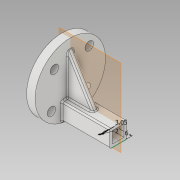
# Autodesk Inventor part: Motor Mount v1
Saved by Autodesk Inventor 2021 (Build 250183000, 183)
## iProperties
Created: 2019-01-09
Part Number: Motor Mount v1
Material: ABS Plastic
Document SubType Name: Modeling
Designer: Kanenas
Density: 1.06 g/cm^3
Appearance: Smooth - White
Mass: 1.86901 g
Surface Area: 21.0001 cm^2
Volume: 1.76322 cm^3
Author: Kanenas
Autodesk Inventor part; units mm, degrees
ref_plane "YZ Plane" through (0, 0, 0) normal (1, 0, 0) x (0, 1, 0)
ref_plane "XZ Plane" through (0, 0, 0) normal (0, 1, 0) x (-1, 0, 0)
sketch "Sketch1" plane through (0, 0, 0) normal (1, 0, 0) x (0, 1, 0)
  line L0 (3.05, 3.05) -> (-3.05, 3.05)
  line L1 (-3.05, 3.05) -> (-3.05, -3.05)
  line L2 (-3.05, -3.05) -> (3.05, -3.05)
  line L3 (3.05, -3.05) -> (3.05, 3.05)
  line L4 (3.05, 3.05) -> (-3.05, -3.05) construction
  line L5 (-3.05, 3.05) -> (3.05, -3.05) construction
  line L6 (2.05, 2.05) -> (-2.05, 2.05)
  line L7 (-2.05, 2.05) -> (-2.05, -2.05)
  line L8 (-2.05, -2.05) -> (2.05, -2.05)
  line L9 (2.05, -2.05) -> (2.05, 2.05)
  line L10 (2.05, 2.05) -> (-2.05, -2.05) construction
  line L11 (-2.05, 2.05) -> (2.05, -2.05) construction
  point P0 (0, 0)
  dimension "d0" = 6.1
  dimension "d1" = 6.1
  dimension "d2" = 4.1
  dimension "d3" = 4.1
  constraints: 24 end point, 4 midpoint, 4 parallel, 2 horizontal, 2 perpendicular
  measures "d0" distance of L2.end L0.start
  measures "d1" distance of L1.end L2.end
  measures "d2" distance of L8.end L6.start
  measures "d3" distance of L7.end L8.end
extrude "Extrusion1" add sketch "Sketch1" along normal blind 20
sketch "Sketch2" plane through (0, 0, 0) normal (-1, 0, 0) x (0, 0, 1)
  circle A0 centre (0, 8.5) radius 12.5
  line L0 (3.05, -3.05) -> (-3.05, -3.05) projected
  line L1 (3.05, -3.05) -> (-3.05, -3.05) projected
  point P0 (0, 0)
  dimension "d6" = 25
  dimension "d8" = 0
  dimension "d63" = 8.5
  constraints: 1 centre point
  measures "d6" diameter of A0
  measures "d8" horizontal distance of point (0, 0) A0.centre
  measures "d63" distance of A0.centre point (0, 0)
extrude "Extrusion2" add sketch "Sketch2" against normal blind 3
sketch "Sketch3" plane through (0, 0, 0) normal (-1, 0, 0) x (0, 0, 1)
  line L0 (-3.05, 3.05) -> (3.05, 3.05)
  line L1 (3.05, 3.05) -> (3.05, -3.05)
  line L2 (3.05, -3.05) -> (-3.05, -3.05)
  line L3 (-3.05, -3.05) -> (-3.05, 3.05)
  line L4 (-3.05, 3.05) -> (3.05, -3.05) construction
  line L5 (3.05, 3.05) -> (-3.05, -3.05) construction
  line L6 (3.05, -3.05) -> (-3.05, -3.05) projected
  line L7 (-3.05, -3.05) -> (-3.05, -2.6722) projected
  point P0 (0, 0)
  constraints: 12 end point, 2 collinear, 2 midpoint, 2 parallel, 1 horizontal, 1 perpendicular
extrude "Extrusion3" add sketch "Sketch3" against normal blind 3
sketch "Sketch4" plane through (0, 0, 0) normal (-1, 0, 0) x (0, 0, 1)
  circle A0 centre (-6.7175, 15.2175) radius 1.5
  line L0 (0, 23.95) -> (0, -8.2808) construction
  circle A1 centre (0, 8.5) radius 9.5 construction
  circle A2 centre (-6.7175, 1.7825) radius 1.5
  circle A3 centre (6.7175, 1.7825) radius 1.5
  circle A4 centre (6.7175, 15.2175) radius 1.5
  line L1 (0, 8.5) -> (9.5, 8.5)
  line L2 (-6.7175, 15.2175) -> (6.7175, 1.7825)
  circle A5 centre (0, 8.5) radius 12.5 projected
  point P0 (0, 0)
  point P1 (-6.4286, 2.2798)
  point P2 (6.4286, 2.2798)
  point P3 (3.05, -2.6722)
  point P4 (-3.05, -2.6722)
  dimension "d17" = 3
  dimension "d22" = 360
  dimension "d29" = 19
  dimension "d30" = 135
  constraints: 6 end point, 5 centre point, 3 point on circle, 1 coincident, 1 horizontal, 1 point on line, 1 vertical, 11 other
  measures "d17" diameter of A0
  measures "d29" diameter of A1
  measures "d30" angle of L2 L1
extrude "Extrusion5" cut sketch "Sketch4" against normal blind 10 contours A0 | A3
sketch "Sketch5" plane through (0, 0, 0) normal (-1, 0, 0) x (0, 0, 1)
  circle A0 centre (0, 8.5) radius 8 construction
  circle A1 centre (0, 8.5) radius 12.5 projected
  circle A2 centre (5.6569, 14.1569) radius 1.5
  line L0 (0, 8.5) -> (0, 19.1117) construction
  line L1 (0, 8.5) -> (15.8394, 8.5) construction
  line L2 (0, 8.5) -> (7.3727, 15.8727) construction
  line L3 (0, 8.5) -> (-7.3727, 1.1273) construction
  circle A3 centre (-5.6569, 2.8431) radius 1.5
  point P0 (0, 0)
  point P1 (-6.4286, 2.2798)
  point P2 (6.4286, 2.2798)
  point P3 (3.05, -2.6722)
  point P4 (-3.05, -2.6722)
  dimension "d33" = 16
  dimension "d34" = 3
  dimension "d35" = 45
  dimension "d38" = 360
  constraints: 8 end point, 2 centre point, 2 point on line, 1 horizontal, 1 vertical, 15 other
  measures "d34" diameter of A2
  measures "d35" angle of L1 L2
extrude "Extrusion6" cut sketch "Sketch5" against normal blind 10 contours A2 | A3
sketch "Sketch8" plane through (0, 0, 0) normal (-1, 0, 0) x (0, 0, 1)
  circle A0 centre (0, 8.5) radius 12.5 projected
  circle A1 centre (0, 8.5) radius 4
  point P0 (0, 0)
  point P1 (-6.4286, 2.2798)
  point P2 (6.4286, 2.2798)
  point P3 (3.05, -2.6722)
  point P4 (-3.05, -2.6722)
  dimension "d52" = 8
  constraints: 1 centre point, 1 coincident, 1 other
  measures "d52" diameter of A1
extrude "Extrusion9" cut sketch "Sketch8" against normal blind 2 contours A1
sketch "Sketch9" plane through (0, -3, 0) normal (0, 0, 1) x (1, 0, 0)
  line L0 (3, 23) -> (3, 11) projected
  line L1 (3, 20.6098) -> (12, 6.05)
  line L2 (3, 6.05) -> (3, 20.6098)
  line L3 (2.5, 11) -> (2.5, 23.5) projected
  line L4 (3, 6.05) -> (12, 6.05)
  line L5 (3, 6.05) -> (20, 6.05) projected
  point P0 (3, 5.7086)
  point P1 (2.5, 5.2798)
  point P2 (3.5, 6.05)
  point P3 (3, 0.9871)
  point P4 (3, 24.45)
  dimension "d62" = 9
  constraints: 6 end point, 1 collinear, 1 parallel, 1 point on line
  measures "d62" horizontal distance of L1.start L1.end
extrude "Extrusion10" add sketch "Sketch9" against normal mid plane 2
fillet "Fillet11" radius 0.5 8 edges at (3, 17.6098, 0) (12, 3.05, 0) (7.5, 10.3299, 1) (7.5, 10.3299, -1) (3, 10.3299, 1) (7.5, 3.05, 1) (7.5, 3.05, -1) (3, 10.3299, -1)
fillet "Fillet12" radius 0.5 4 edges at (11.5, 3.05, 3.05) (11.5, -3.05, 3.05) (11.5, 3.05, -3.05) (11.5, -3.05, -3.05)
fillet "Fillet13" radius 0.5 11 edges at (3, -2.9036, 2.9036) (3, -3.05, 0) (3, -2.9036, -2.9036) (3, 0, -3.05) (3, 2.9036, -2.9036) (3, 3.05, -2.025) (3.1464, 3.1964, -1.1464) (3, 2.9036, 2.9036) (3, 3.05, 2.025) (3.1464, 3.1964, 1.1464) (3, 0, 3.05)
sketch "Sketch10" plane through (20, -3.05, -2.55) normal (0, -1, 0) x (1, 0, 0)
  circle A0 centre (-6, 2.55) radius 1
  line L0 (-16.5, -0.5) -> (0, -0.5) projected
  line L1 (0, 5.1) -> (0, 0) projected
  point P0 (-20, 2.55)
  dimension "d66" = 2
  dimension "d67" = 3.05
  dimension "d68" = 6
  constraints: 1 centre point
  measures "d66" diameter of A0
  measures "d67" distance from line of L0 A0.centre
  measures "d68" distance from line of L1 A0.centre
body "Solid1"
